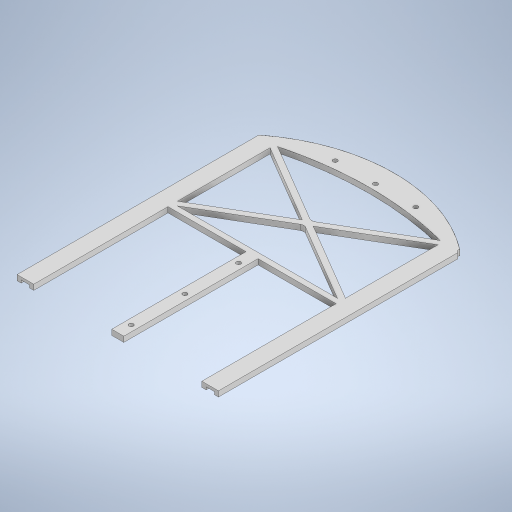
# Autodesk Inventor part: お盆4
Saved by Autodesk Inventor 2023 (Build 270158000, 158)
## iProperties
Created: 2022-12-03
Part Number: お盆4
Material: 一般
Document SubType Name: Modeling
Designer: RiSA
Density: 1 g/cm^3
Appearance: 既定
Author: RiSA
Autodesk Inventor part; units mm, degrees
ref_plane "YZ Plane" through (0, 0, 0) normal (1, 0, 0) x (0, 1, 0)
ref_plane "XZ Plane" through (0, 0, 0) normal (0, 1, 0) x (-1, 0, 0)
ref_plane "XY Plane" through (0, 0, 0) normal (0, 0, 1) x (1, 0, 0)
sketch "スケッチ1" plane through (0, 0, 0) normal (0, 1, 0) x (-1, 0, 0)
  line L0 (-75, -90) -> (75, -90)
  line L1 (75, -90) -> (75, 90)
  line L2 (75, 90) -> (-75, 90)
  line L3 (-75, 90) -> (-75, -90)
  line L4 (-75, -90) -> (75, 90) construction
  line L5 (75, -90) -> (-75, 90) construction
  point P0 (0, 0)
  dimension "d0" = 150
  dimension "d1" = 180
  constraints: 12 end point, 2 midpoint, 2 parallel, 1 horizontal, 1 perpendicular
  measures "d0" distance of L2.end L1.end
  measures "d1" distance of L1.end L0.end
extrude "押し出し1" add sketch "スケッチ1" along normal blind 4
sketch "スケッチ2" plane through (0, 4, 0) normal (0, 1, 0) x (1, 0, 0)
  line L0 (-75, -90) -> (75, -90) projected
  line L1 (-62.6, -90) -> (62.6, -90)
  line L2 (62.6, -90) -> (62.6, 10)
  line L3 (62.6, 10) -> (-62.6, 10)
  line L4 (-62.6, 10) -> (-62.6, -90)
  point P0 (0, 0)
  dimension "d4" = 125.2
  dimension "d5" = 100
  dimension "d6" = 62.6
  constraints: 8 end point, 2 parallel, 1 horizontal, 1 perpendicular, 1 point on line
  measures "d4" distance of L3.end L2.end
  measures "d5" distance of L2.end L1.end
  measures "d6" distance from line of point (0, 0) L4
extrude "押し出し2" cut sketch "スケッチ2" against normal blind 4
sketch "スケッチ3" plane through (0, 0, 0) normal (0, -1, 0) x (1, 0, 0)
  line L0 (62.6, 90) -> (75, 90) projected
  line L1 (72, 90) -> (65.8, 90)
  line L2 (65.8, 90) -> (65.8, -90)
  line L3 (65.8, -90) -> (72, -90)
  line L4 (72, -90) -> (72, 90)
  line L5 (75, 90) -> (75, -90) projected
  line L6 (0, 0) -> (0, 35.088)
  line L7 (-62.6, 90) -> (-75, 90)
  line L8 (-72, 90) -> (-65.8, 90)
  line L9 (-65.8, 90) -> (-65.8, -90)
  line L10 (-65.8, -90) -> (-72, -90)
  line L11 (-72, -90) -> (-72, 90)
  line L12 (-75, 90) -> (-75, -90)
  dimension "d9" = 6.2
  dimension "d10" = 180
  dimension "d11" = 3
  constraints: 22 end point, 7 symmetric about line, 2 parallel, 2 point on line, 1 horizontal, 1 perpendicular, 1 vertical
  measures "d9" distance of L3.end L2.end
  measures "d10" distance of L2.end L1.end
  measures "d11" distance between parallel lines of L5 L4
extrude "押し出し3" cut sketch "スケッチ3" against normal blind 2
sketch "スケッチ4" plane through (0, 4, 0) normal (0, 1, 0) x (1, 0, 0)
  line L0 (62.6, 10) -> (-62.6, 10) projected
  line L1 (-4.5, 10) -> (4.5, 10)
  line L2 (4.5, 10) -> (4.5, -90)
  line L3 (4.5, -90) -> (-4.5, -90)
  line L4 (-4.5, -90) -> (-4.5, 10)
  point P0 (0, 0)
  dimension "d14" = 9
  dimension "d15" = 100
  dimension "d16" = 4.5
  constraints: 8 end point, 2 parallel, 1 horizontal, 1 perpendicular, 1 point on line
  measures "d14" distance of L2.end L3.end
  measures "d15" distance of L1.end L2.end
  measures "d16" distance from line of point (0, 0) L4
extrude "押し出し4" add sketch "スケッチ4" against normal blind 4
sketch "スケッチ5" plane through (0, 4, 0) normal (0, 1, 0) x (1, 0, 0)
  circle A0 centre (0, -5.589) radius 121.5
  line L0 (75, 90) -> (72, 90) projected
  line L1 (-75, 90) -> (-75, -90) projected
  line L2 (-75, 90) -> (75, 90)
  point P0 (0, 0)
  dimension "d19" = 243
  constraints: 2 end point, 2 point on circle, 1 centre point, 1 horizontal
  measures "d19" diameter of A0
extrude "押し出し5" add sketch "スケッチ5" against normal blind 4 contours L0 L2 A0 picked at (-21.9725, 92.7838)
sketch "スケッチ6" plane through (0, 4, 0) normal (0, 1, 0) x (1, 0, 0)
  arc A0 (75, 90) -> (-75, 90) centre (0, -5.589) ccw projected
  line L0 (75, 90) -> (-75, 90) construction
  line L1 (0, 90) -> (0, 115.911) construction
  point P0 (0, 0)
  point P1 (0, 102)
  point P2 (30, 102)
  point P3 (-30, 102)
  dimension "d22" = 12
  dimension "d23" = 30
  constraints: 4 end point, 1 midpoint, 1 point on circle, 1 point on line, 1 symmetric about line
  measures "d22" distance from line of point (0, 102) L0
  measures "d23" distance of point (30, 102) point (0, 102)
hole "穴1" at (75, 4, -90) at (0, 4, -102) at (30, 4, -102) at (-30, 4, -102) direction (0, -1, 0) diameter 3.2 end through all
sketch "スケッチ7" plane through (0, 4, 0) normal (0, 1, 0) x (1, 0, 0)
  line L0 (-62.6, 10) -> (-4.5, 10) projected
  line L1 (-62.6, 14) -> (62.6, 14)
  line L2 (62.6, 14) -> (62.6, 89)
  line L3 (-62.6, 89) -> (-62.6, 14)
  arc A0 (62.6, 89) -> (-62.6, 89) centre (0, -137.2653) ccw
  line L4 (-59.6, 14) -> (62.6, 86)
  line L5 (-62.6, 17) -> (60.547, 89.558)
  line L6 (0, 14) -> (0, 41.0158)
  line L7 (59.6, 14) -> (-62.6, 86)
  line L8 (62.6, 17) -> (-60.547, 89.558)
  point P0 (0, 0)
  point P1 (0, 97.5)
  point P2 (0, 53.8838)
  point P3 (-4.0458, 51.5)
  point P4 (0, 49.1162)
  point P5 (4.0458, 51.5)
  dimension "d32" = 4
  dimension "d33" = 125.2
  dimension "d34" = 75
  dimension "d36" = 3
  dimension "d37" = 3
  dimension "d38" = 3
  constraints: 16 end point, 4 point on circle, 4 symmetric about line, 3 point on line, 2 parallel, 1 centre point, 1 horizontal, 1 midpoint, 1 perpendicular, 1 vertical
  measures "d32" distance from line of L1.start L0
  measures "d33" distance of L3.start L2.end
  measures "d34" distance of L2.end L1.end
  measures "d36" distance from line of L3 L4.start
  measures "d37" distance from line of L5.start L1
  measures "d38" distance of L2.end L4.end
extrude "押し出し6" cut sketch "スケッチ7" against normal blind 4 contours L4 L7 L1 | L3 L7 L5 | L4 L2 L8 | L8 A0 L5
sketch "スケッチ8" plane through (0, 4, 0) normal (0, 1, 0) x (1, 0, 0)
  line L0 (-62.6, 10) -> (-4.5, 10) projected
  point P0 (0, 0)
  point P1 (0, 0)
  point P2 (0, -40)
  point P3 (0, -80)
  dimension "d41" = 10
  dimension "d42" = 50
  dimension "d43" = 90
  measures "d41" distance from line of point (0, 0) L0
  measures "d42" distance from line of point (0, -40) L0
  measures "d43" distance from line of point (0, -80) L0
hole "穴2" at (0, 4, 0) at (0, 4, 40) at (0, 4, 80) direction (0, -1, 0) diameter 3.2 end through all
fillet "フィレット1" radius 4 2 edges at (0, 2, -49.1162) (0, 2, -53.8838)
